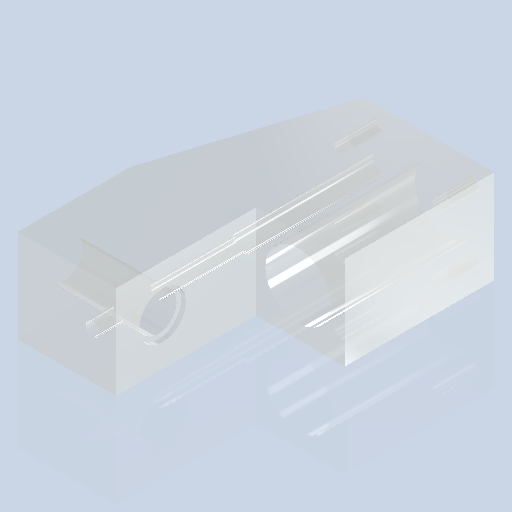
# Autodesk Inventor part: MotorBlock
Saved by Autodesk Inventor 2024.2 (Build 282272000, 272)
## iProperties
Created: 2024-01-15
Part Number: MotorBlock
Material: Glas
Document SubType Name: Modeling
Designer: ffogue
Density: 2.18 g/cm^3
Appearance: Klar
Author: ffogue
Autodesk Inventor part; units mm, degrees
note: some values were not read from the file. Chosen so that the rebuilt part matches the saved one: direction of "Bohrung3"; direction of "Bohrung4".
ref_plane "XY Plane" through (0, 0, 0) normal (0, 0, 1) x (1, 0, 0)
sketch "Skizze1" plane through (0, 0, 0) normal (0, 0, 1) x (1, 0, 0)
  line L0 (0, 0) -> (0, 24)
  line L1 (0, 24) -> (12, 62)
  line L2 (12, 62) -> (40, 62)
  line L3 (40, 62) -> (40, 30)
  line L4 (40, 30) -> (21, 30)
  line L5 (21, 30) -> (21, 0)
  line L6 (21, 0) -> (0, 0)
  dimension "d0" = 62
  dimension "d1" = 21
  dimension "d2" = 30
  dimension "d3" = 38
  dimension "d4" = 28
  dimension "d5" = 12
  constraints: 14 end point, 3 perpendicular, 2 parallel, 1 coincident, 1 vertical
  measures "d0" distance between parallel lines of L6 L2
  measures "d1" distance between parallel lines of L5 L0
  measures "d2" distance between parallel lines of L6 L4
  measures "d3" distance from line of L2 L0.end
  measures "d4" distance of L2.end L1.end
  measures "d5" horizontal distance of L1.end L0.end
extrude "Extrusion1" add sketch "Skizze1" along normal blind 20
sketch "Skizze3" plane through (12, 62, 0) normal (0, 1, 0) x (1, 0, 0)
  line L0 (0, 0) -> (0, -20) projected
  line L1 (28, 0) -> (28, -20) projected
  point P0 (-12, 0)
  point P1 (18, -10)
  point P2 (28, -10)
  dimension "d16" = 10
  constraints: 1 horizontal alignment, 1 midpoint
  measures "d16" distance from line of L1 point (18, -10)
hole "Bohrung2" at (30, 62, 10) direction (0, -1, 0) diameter 14 end through all
sketch "Skizze4" plane through (12, 62, 0) normal (0, 1, 0) x (1, 0, 0)
  line L0 (0, 0) -> (0, -20) projected
  line L1 (28, 0) -> (28, -20) projected
  point P0 (-12, 0)
  point P1 (4, -10)
  point P2 (28, -10)
  dimension "d24" = 4
  constraints: 1 horizontal alignment, 1 midpoint
  measures "d24" distance from line of point (4, -10) L0
hole "Bohrung3" at (16, 62, 10) direction (0, -1, 0) diameter 3 depth 62 counterbore diameter 4 counterbore depth 30
sketch "Skizze5" plane through (21, 0, 0) normal (1, 0, 0) x (0, 0, -1)
  line L0 (0, 0) -> (-20, 0) projected
  point P0 (-10, 10)
  point P1 (-10, 0)
  dimension "d32" = 10
  constraints: 1 midpoint, 1 vertical alignment
  measures "d32" distance from line of L0 point (-10, 10)
hole "Bohrung4" at (21, 10, 10) direction (-1, 0, 0) diameter 8 depth 21 counterbore diameter 10 counterbore depth 1
ref_plane "Arbeitsebene1" through (0, 12, 0) normal (0, 1, 0) x (-1, 0, 0)
sketch "Skizze8" plane through (12, 62, 0) normal (0, 1, 0) x (1, 0, 0)
  circle A0 centre (4, -10) radius 2 projected
  circle A1 centre (18, -10) radius 7 projected
  line L0 (28, 0) -> (0, 0) projected
  line L1 (0, 0) -> (0, -20) projected
  line L2 (28, -20) -> (0, -20) projected
  line L3 (28, 0) -> (28, -20) projected
  line L4 (4, -10) -> (4, -3) construction
  line L5 (4, -10) -> (4, -17) construction
  line L6 (18, -10) -> (9, -10) construction
  line L7 (9, 0) -> (9, -20) projected
  point P0 (-12, 0)
  dimension "d57" = 14
  constraints: 6 end point, 2 vertical, 1 midpoint, 1 symmetric about line
  measures "d57" distance of L4.end L5.end
hole "Bohrung7" at (16, 62, 17) at (16, 62, 3) direction (0, -1, 0) diameter 2.459 depth 9 tip angle 118 thread size "M3x0.5" class "6H" standard "ISO Metric profile"
ref_plane "Arbeitsebene2" through (26.5, 0, 0) normal (1, 0, 0) x (0, 1, 0)
mirror "Spiegeln2" about plane through (26.5, 0, 0) normal (1, 0, 0) of "Bohrung7"
